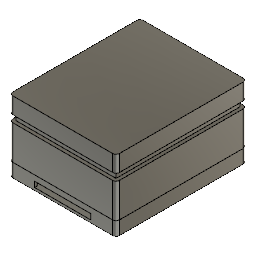
Weave pedal v9 (Autodesk Fusion 360 design; units mm, degrees)
Autodesk Fusion 360 part; units mm, degrees
note: some values were not read from the file. Chosen so that the rebuilt part matches the saved one: which bodies a step acts on; which face or edge a step refers to.
sketch "Sketch1" plane through (0, 0, 0) normal (0, 0, 1) x (1, 0, 0)
  line L0 (39, 47.75) -> (-39, 47.75)
  line L1 (-39, 47.75) -> (-39, -47.75)
  line L2 (-39, -47.75) -> (39, -47.75)
  line L3 (39, -47.75) -> (39, 47.75)
  line L4 (39, 47.75) -> (-39, -47.75) construction
  line L5 (-39, 47.75) -> (39, -47.75) construction
  dimension "d1" = 78
  dimension "d2" = 95.5
  constraint horizontal L0
  constraint perpendicular L0 L1
  constraint parallel L0 L2
  constraint parallel L1 L3
  constraint coincident L4 origin
  constraint coincident L5 origin
  measures "d1" distance of L1.end L2.end
  measures "d2" distance of L0.end L1.end
sketch "Sketch3" plane through (0, 0, 0) normal (1, 0, 0) x (0, 1, 0)
  line L0 (-55, 10) -> (55, 10)
  constraint horizontal L0
extrude "Extrude1" add sketch "Sketch1" along normal blind 35 makes body 1
fillet "Fillet1" radius 2.5 4 edges at (39, -47.75, 17.5) (-39, -47.75, 17.5) (39, 47.75, 17.5) (-39, 47.75, 17.5) on bodies 1
split "Split1" by curves path "Sketch3" along L0 bodies 1 makes body 2 at (-13, 15.0833, 0)
sketch "Sketch4" plane through (0, 0, 35) normal (0, 0, 1) x (-1, 0, 0)
  arc A0 (36.5, -47.75) -> (39, -45.25) centre (36.5, -45.25) ccw
  line L0 (39, -45.25) -> (39, 45.25)
  arc A1 (39, 45.25) -> (36.5, 47.75) centre (36.5, 45.25) ccw
  line L1 (36.5, 47.75) -> (-36.5, 47.75)
  arc A2 (-36.5, 47.75) -> (-39, 45.25) centre (-36.5, 45.25) ccw
  line L2 (-39, 45.25) -> (-39, -45.25)
  arc A3 (-39, -45.25) -> (-36.5, -47.75) centre (-36.5, -45.25) ccw
  line L3 (-36.5, -47.75) -> (36.5, -47.75)
  line L4 (36.5, -45.25) -> (36.5, 45.25)
  line L5 (36.5, 45.25) -> (-36.5, 45.25)
  line L6 (-36.5, 45.25) -> (-36.5, -45.25)
  line L7 (-36.5, -45.25) -> (36.5, -45.25)
  line L8 (34, -42.75) -> (34, 42.75)
  line L9 (34, 42.75) -> (-34, 42.75)
  line L10 (-34, 42.75) -> (-34, -42.75)
  line L11 (-34, -42.75) -> (34, -42.75)
  dimension "d7" = -2.5
  dimension "d8" = -5
extrude "Extrude2" add sketch "Sketch4" along normal blind 10 separate body contours L4 L5 L6 L7 makes body 3
sketch "Sketch5" plane through (0, 0, 35) normal (0, 0, 1) x (-1, 0, 0)
  circle A0 centre (0, 0) radius 5.75
  arc A1 (36.5, -47.75) -> (39, -45.25) centre (36.5, -45.25) ccw
  line L0 (39, -45.25) -> (39, 45.25)
  arc A2 (39, 45.25) -> (36.5, 47.75) centre (36.5, 45.25) ccw
  line L1 (36.5, 47.75) -> (-36.5, 47.75)
  arc A3 (-36.5, 47.75) -> (-39, 45.25) centre (-36.5, 45.25) ccw
  line L2 (-39, 45.25) -> (-39, -45.25)
  arc A4 (-39, -45.25) -> (-36.5, -47.75) centre (-36.5, -45.25) ccw
  line L3 (-36.5, -47.75) -> (36.5, -47.75)
  dimension "d11" = 11.5
  constraint coincident A0.centre origin
  measures "d11" diameter of A0
shell "Shell1" thickness 2 removed faces 1 at (13, -15.0833, 10) on bodies 1
shell "Shell2" thickness 2 removed faces 1 at (13, -15.0833, 10) on bodies 2
extrude "Extrude3" cut sketch "Sketch5" against normal blind 5 contours A0 bodies 1
sketch "Sketch6" plane through (0, 0, 2) normal (0, 0, 1) x (-1, 0, 0)
  arc A0 (36.5, -45.75) -> (37, -45.25) centre (36.5, -45.25) ccw
  line L0 (37, -45.25) -> (37, 45.25)
  arc A1 (37, 45.25) -> (36.5, 45.75) centre (36.5, 45.25) ccw
  line L1 (36.5, 45.75) -> (-36.5, 45.75)
  arc A2 (-36.5, 45.75) -> (-37, 45.25) centre (-36.5, 45.25) ccw
  line L2 (-37, 45.25) -> (-37, -45.25)
  arc A3 (-37, -45.25) -> (-36.5, -45.75) centre (-36.5, -45.25) ccw
  line L3 (-36.5, -45.75) -> (36.5, -45.75)
  line L4 (-37, -39.75) -> (-34, -39.75)
  line L5 (-34, -39.75) -> (-34, -32.25)
  line L6 (-34, -32.25) -> (-37, -32.25)
  line L7 (-37, -32.25) -> (-37, -39.75)
  line L8 (37, -39.75) -> (34, -39.75)
  line L9 (34, -39.75) -> (34, -32.25)
  line L10 (34, -32.25) -> (37, -32.25)
  line L11 (37, -32.25) -> (37, -39.75)
  line L12 (37, 39.75) -> (34, 39.75)
  line L13 (34, 39.75) -> (34, 32.25)
  line L14 (34, 32.25) -> (37, 32.25)
  line L15 (37, 32.25) -> (37, 39.75)
  line L16 (-37, 39.75) -> (-34, 39.75)
  line L17 (-34, 39.75) -> (-34, 32.25)
  line L18 (-34, 32.25) -> (-37, 32.25)
  line L19 (-37, 32.25) -> (-37, 39.75)
  dimension "d16" = 3
  dimension "d17" = 7.5
  dimension "d18" = 6
  dimension "d19" = 3
  dimension "d20" = 7.5
  dimension "d21" = 6
  dimension "d22" = 3
  dimension "d23" = 7.5
  dimension "d24" = 6
  dimension "d25" = 3
  dimension "d26" = 7.5
  dimension "d27" = 6
  constraint horizontal L4
  constraint vertical L5
  constraint horizontal L6
  constraint vertical L7
  constraint coincident L2 L4.start
  constraint horizontal L8
  constraint vertical L9
  constraint horizontal L10
  constraint vertical L11
  constraint coincident L0 L8.start
  constraint horizontal L12
  constraint vertical L13
  constraint horizontal L14
  constraint vertical L15
  constraint coincident L0 L12.start
  constraint horizontal L16
  constraint vertical L17
  constraint horizontal L18
  constraint vertical L19
  constraint coincident L2 L16.start
  measures "d16" distance of L4.start L4.end
  measures "d17" distance of L4.start L6.end
  measures "d18" distance of L3 L4
  measures "d19" distance of L8.start L8.end
  measures "d20" distance of L8.start L10.end
  measures "d21" distance of L3 L8
  measures "d22" distance of L12.start L12.end
  measures "d23" distance of L12.start L14.end
  measures "d24" distance of L1 L12
  measures "d25" distance of L16.start L16.end
  measures "d26" distance of L16.start L18.end
  measures "d27" distance of L1 L16
extrude "Extrude4" add sketch "Sketch6" along normal blind 12 contours L0 L8 L9 L10 L11 | L2 L4 L5 L6 L7 | L0 L12 L13 L14 L15 | L2 L16 L17 L18 L19 bodies 2
sketch "Sketch9" plane through (0, -47.75, 0) normal (0, -1, 0) x (1, 0, 0)
  line L0 (36.5, 10) -> (-36.5, 10)
  line L1 (-36.5, 10) -> (-36.5, 0)
  line L2 (-36.5, 0) -> (36.5, 0)
  line L3 (36.5, 0) -> (36.5, 10)
  line L4 (20.5, 6) -> (-20.5, 6)
  line L5 (-20.5, 6) -> (-20.5, 2)
  line L6 (-20.5, 2) -> (20.5, 2)
  line L7 (20.5, 2) -> (20.5, 6)
  line L8 (20.5, 6) -> (-20.5, 2) construction
  line L9 (-20.5, 6) -> (20.5, 2) construction
  point P0 (0, 4)
  dimension "d30" = 41
  dimension "d31" = 4
  dimension "d33" = 6
  dimension "d34" = 16
  constraint horizontal L4
  constraint perpendicular L4 L5
  constraint parallel L4 L6
  constraint parallel L5 L7
  constraint coincident L8 P0
  constraint coincident L9 P0
  measures "d30" distance of L5.end L6.end
  measures "d31" distance of L4.end L5.end
  measures "d33" distance of L2 L4
  measures "d34" distance of L3 L7
extrude "Extrude5" cut sketch "Sketch9" against normal blind 15 contours L4 L5 L6 L7 bodies 2
sketch "Sketch10" plane through (0, 47.75, 0) normal (0, 1, 0) x (-1, 0, 0)
  line L0 (36.5, 10) -> (-36.5, 10)
  line L1 (-36.5, 10) -> (-36.5, 0)
  line L2 (-36.5, 0) -> (36.5, 0)
  line L3 (36.5, 0) -> (36.5, 10)
  line L4 (21.5, 2) -> (-21.5, 2)
  line L5 (-21.5, 2) -> (-21.5, 6.5)
  line L6 (-21.5, 6.5) -> (21.5, 6.5)
  line L7 (21.5, 6.5) -> (21.5, 2)
  line L8 (21.5, 2) -> (-21.5, 6.5) construction
  line L9 (-21.5, 2) -> (21.5, 6.5) construction
  point P0 (0, 4.25)
  dimension "d37" = 43
  dimension "d38" = 4.5
  dimension "d40" = 2
  dimension "d41" = 15
  constraint horizontal L4
  constraint perpendicular L4 L5
  constraint parallel L4 L6
  constraint parallel L5 L7
  constraint coincident L8 P0
  constraint coincident L9 P0
  measures "d37" distance of L5.end L6.end
  measures "d38" distance of L4.end L5.end
  measures "d40" distance of L2 L4
  measures "d41" distance of L3 L7
extrude "Extrude6" cut sketch "Sketch10" against normal blind 10 contours L4 L5 L6 L7 bodies 2
ref_plane "WorkPlane1" through (0, 0, 40) normal (0, 0, 1) x (1, 0, 0)
sketch "Sketch11" plane through (0, 0, 40) normal (0, 0, 1) x (1, 0, 0)
  line L0 (39, -47.75) -> (-39, -47.75)
  line L1 (-39, -47.75) -> (-39, 47.75)
  line L2 (-39, 47.75) -> (39, 47.75)
  line L3 (39, 47.75) -> (39, -47.75)
  line L4 (39, -47.75) -> (-39, 47.75) construction
  line L5 (-39, -47.75) -> (39, 47.75) construction
  dimension "d45" = 78
  dimension "d46" = 95.5
  constraint horizontal L0
  constraint perpendicular L0 L1
  constraint parallel L0 L2
  constraint parallel L1 L3
  constraint coincident L4 origin
  constraint coincident L5 origin
  measures "d45" distance of L1.end L2.end
  measures "d46" distance of L0.end L1.end
extrude "Extrude7" add sketch "Sketch11" along normal blind 12 separate body makes body 4
fillet "Fillet2" radius 2.5 4 edges at (39, -47.75, 46) (-39, -47.75, 46) (39, 47.75, 46) (-39, 47.75, 46) on bodies 4
shell "Shell3" thickness 1.7 removed faces 1 at (-13, 15.0833, 40) on bodies 4
sketch "Sketch12" plane through (0, 0, 50.3) normal (0, 0, -1) x (1, 0, 0)
  arc A0 (-37.3, -45.25) -> (-36.5, -46.05) centre (-36.5, -45.25) ccw
  line L0 (-36.5, -46.05) -> (36.5, -46.05)
  arc A1 (36.5, -46.05) -> (37.3, -45.25) centre (36.5, -45.25) ccw
  line L1 (37.3, -45.25) -> (37.3, 45.25)
  arc A2 (37.3, 45.25) -> (36.5, 46.05) centre (36.5, 45.25) ccw
  line L2 (36.5, 46.05) -> (-36.5, 46.05)
  arc A3 (-36.5, 46.05) -> (-37.3, 45.25) centre (-36.5, 45.25) ccw
  line L3 (-37.3, 45.25) -> (-37.3, -45.25)
  circle A4 centre (0, 0) radius 6
  circle A5 centre (0, 0) radius 8
  dimension "d52" = 12
  dimension "d53" = 2
  constraint coincident A4.centre A5.centre
  measures "d52" diameter of A4
extrude "Extrude8" add sketch "Sketch12" along normal blind 5 contours A5 bodies 4
named bodies: "Top piece", "bottom piece", "Pedal"
